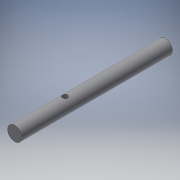
# Autodesk Inventor part: axle
Saved by Autodesk Inventor 2017 (Build 210142000, 142)
## iProperties
Created: 2018-11-23
Part Number: axle
Material: Generic
Document SubType Name: Modeling
Designer: Eric the Great
Density: 1 g/cm^3
Appearance: Default
Author: Eric the Great
Autodesk Inventor part; units mm, degrees
ref_plane "YZ Plane" through (0, 0, 0) normal (1, 0, 0) x (0, 1, 0)
ref_plane "XZ Plane" through (0, 0, 0) normal (0, 1, 0) x (-1, 0, 0)
ref_plane "XY Plane" through (0, 0, 0) normal (0, 0, 1) x (1, 0, 0)
sketch "Sketch1" plane through (0, 0, 0) normal (0, 0, 1) x (1, 0, 0)
  circle A0 centre (0, 0) radius 4
  dimension "d0" = 8
  constraints: 1 centre point, 1 coincident
  measures "d0" diameter of A0
extrude "Extrusion1" add sketch "Sketch1" along normal blind 84
sketch "Sketch2" plane through (0, 0, 0) normal (0, 1, 0) x (-1, 0, 0)
  circle A0 centre (0, 56) radius 1.5
  line L0 (4, 84) -> (-4, 84) projected
  line L1 (-4, 0) -> (4, 0) projected
  point P0 (0, 0)
  dimension "d3" = 3
  dimension "d7" = 56
  constraints: 1 centre point
  measures "d3" diameter of A0
  measures "d7" distance from line of L1 A0.centre
extrude "Extrusion2" cut sketch "Sketch2" along normal mid plane 100
body "Solid1"
